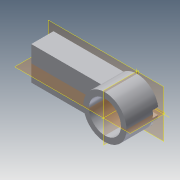
# Autodesk Inventor part: HbThumbProximalPhalanx01
Saved by Autodesk Inventor 2015 SP1 (Build 190203100, 203)
## iProperties
Created: 2015-09-12
Part Number: HbThumbProximalPhalanx01
Material: ABS プラスチック
Document SubType Name: Modeling
Designer: Yamaura
Density: 1.06 g/cm^3
Appearance: 滑らか - 白
Author: Yamaura
Autodesk Inventor part; units mm, degrees
sketch "スケッチ1" plane through (0, 0, 0) normal (0, 0, 1) x (1, 0, 0)
  circle A0 centre (0, 0) radius 5.75
  circle A1 centre (0, 0) radius 7.75
  dimension "d0" = 11.5
  dimension "d1" = 15.5
  constraints: 2 centre point, 2 coincident
  measures "d0" diameter of A0
  measures "d1" diameter of A1
extrude "押し出し1" add sketch "スケッチ1" along normal blind 11.5 contours A0 | A1
sketch "スケッチ2" plane through (0, 0, 0) normal (0, 0, 1) x (1, 0, 0)
  line L0 (-30, 6) -> (0, 6)
  line L1 (0, 6) -> (0, -6)
  line L2 (0, -6) -> (-30, -6)
  line L3 (-30, -6) -> (-30, 6)
  point P0 (0, 0)
  dimension "d4" = 30
  dimension "d5" = 6
  dimension "d6" = 12
  constraints: 8 end point, 2 parallel, 1 horizontal, 1 midpoint, 1 perpendicular
  measures "d4" distance from line of L3 point (0, 0)
  measures "d5" distance from line of L0 point (0, 0)
  measures "d6" distance of L2.end L0.start
extrude "押し出し2" add sketch "スケッチ2" along normal blind 8
sketch "スケッチ3" plane through (0, 0, 0) normal (0, 0, 1) x (1, 0, 0)
  circle A0 centre (0, 0) radius 5.75
  dimension "d9" = 11.5
  constraints: 1 centre point, 1 coincident
  measures "d9" diameter of A0
extrude "押し出し3" cut sketch "スケッチ3" along normal blind 11.5
sketch "スケッチ4" plane through (0, 0, 0) normal (0, 0, 1) x (1, 0, 0)
  line L0 (-8.5, 1.25) -> (8.5, 1.25)
  line L1 (8.5, 1.25) -> (8.5, -1.25)
  line L2 (8.5, -1.25) -> (-8.5, -1.25)
  line L3 (-8.5, -1.25) -> (-8.5, 1.25)
  line L4 (-8.5, 1.25) -> (8.5, -1.25) construction
  line L5 (8.5, 1.25) -> (-8.5, -1.25) construction
  point P0 (0, 0)
  dimension "d12" = 17
  dimension "d13" = 2.5
  constraints: 12 end point, 2 midpoint, 2 parallel, 1 horizontal, 1 perpendicular
  measures "d12" distance of L1.end L2.end
  measures "d13" distance of L0.end L1.end
extrude "押し出し4" cut sketch "スケッチ4" along normal blind 2
pattern_circular "円形状パターン1" count 2 over 30 about axis through (0, 0, -10) along (0, 0, -1) of "押し出し4"
